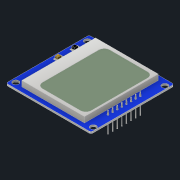
# Autodesk Inventor part: Nokia LCD
Saved by Autodesk Inventor 2022 (Build 260153000, 153)
## iProperties
Created: 2020-05-12
Part Number: Nokia LCD
Material: Generic
Document SubType Name: Modeling
Designer: Arrofiq
Density: 1 g/cm^3
Appearance: Aluminum - Polished
Author: Arrofiq
Autodesk Inventor part; units mm, degrees
ref_plane "YZ Plane" through (0, 0, 0) normal (1, 0, 0) x (0, 1, 0)
ref_plane "XZ Plane" through (0, 0, 0) normal (0, 1, 0) x (-1, 0, 0)
ref_plane "XY Plane" through (0, 0, 0) normal (0, 0, 1) x (1, 0, 0)
sketch "Sketch1" plane through (0, 0, 0) normal (0, 1, 0) x (-1, 0, 0)
  line L0 (23, -22.5) -> (-23, -22.5)
  line L1 (-23, -22.5) -> (-23, 22.5)
  line L2 (-23, 22.5) -> (23, 22.5)
  line L3 (23, 22.5) -> (23, -22.5)
  line L4 (23, -22.5) -> (-23, 22.5) construction
  line L5 (-23, -22.5) -> (23, 22.5) construction
  point P0 (0, 0)
  dimension "d0" = 46
  dimension "d1" = 45
  constraints: 12 end point, 2 midpoint, 2 parallel, 1 horizontal, 1 perpendicular
  measures "d0" distance of L1.end L2.end
  measures "d1" distance of L0.end L1.end
extrude "Extrusion1" add sketch "Sketch1" along normal mid plane 1
sketch "Sketch2" plane through (0, 0.5, 0) normal (0, 1, 0) x (1, 0, 0)
  line L0 (-17, 20) -> (17, 20)
  line L1 (17, 20) -> (17, -20)
  line L2 (17, -20) -> (-17, -20)
  line L3 (-17, -20) -> (-17, 20)
  line L4 (-17, 20) -> (17, -20) construction
  line L5 (17, 20) -> (-17, -20) construction
  line L6 (23, -22.5) -> (23, 22.5) projected
  line L7 (-23, 22.5) -> (-23, -22.5) projected
  point P0 (0, 0)
  point P1 (0, 0)
  point P2 (0, 0)
  dimension "d4" = 34
  dimension "d5" = 40
  dimension "d8" = 6
  dimension "d9" = 6
  constraints: 12 end point, 3 midpoint, 2 parallel, 1 coincident, 1 horizontal, 1 perpendicular
  measures "d4" distance of L1.end L2.end
  measures "d5" distance of L0.end L1.end
  measures "d8" distance between parallel lines of L6 L1
  measures "d9" distance between parallel lines of L7 L3
extrude "Extrusion2" add sketch "Sketch2" along normal blind 3
sketch "Sketch3" plane through (0, 3.5, 0) normal (0, 1, 0) x (1, 0, 0)
  line L0 (-10.5, 18.25) -> (16, 18.25)
  line L1 (16, 18.25) -> (16, -18.25)
  line L2 (16, -18.25) -> (-10.5, -18.25)
  line L3 (-10.5, -18.25) -> (-10.5, 18.25)
  line L4 (-10.5, 18.25) -> (16, -18.25) construction
  line L5 (16, 18.25) -> (-10.5, -18.25) construction
  line L6 (17, -20) -> (17, 20) projected
  point P0 (2.75, 0)
  dimension "d10" = 26.5
  dimension "d11" = 36.5
  dimension "d13" = 1
  constraints: 12 end point, 2 midpoint, 2 parallel, 1 horizontal, 1 perpendicular
  measures "d10" distance of L1.end L2.end
  measures "d11" distance of L0.end L1.end
  measures "d13" distance between parallel lines of L6 L1
extrude "Extrusion3" cut sketch "Sketch3" against normal blind 0.05
sketch "Sketch4" plane through (0, 0.5, 0) normal (0, 1, 0) x (1, 0, 0)
  circle A0 centre (21.3, 19.3) radius 1.6
  line L0 (23, 22.5) -> (-23, 22.5) projected
  line L1 (23, -22.5) -> (23, 22.5) projected
  circle A1 centre (-20.7, 19.3) radius 1.6
  line L2 (-23, 22.5) -> (-23, -22.5) projected
  circle A2 centre (-20.7, -19.5) radius 1.6
  line L3 (-23, -22.5) -> (23, -22.5) projected
  circle A3 centre (21.3, -19.5) radius 1.6
  point P0 (0, 0)
  dimension "d16" = 3.2
  dimension "d19" = 3.2
  dimension "d22" = 3.2
  dimension "d23" = 2.3
  dimension "d24" = 3
  dimension "d25" = 3.2
  dimension "d84" = 38.8
  dimension "d85" = 42
  constraints: 4 centre point, 2 horizontal alignment, 2 vertical alignment
  measures "d16" diameter of A0
  measures "d19" diameter of A1
  measures "d22" diameter of A2
  measures "d23" distance from line of L2 A2.centre
  measures "d24" distance from line of L3 A2.centre
  measures "d25" diameter of A3
  measures "d84" distance of A1.centre A2.centre
  measures "d85" distance of A2.centre A3.centre
extrude "Extrusion4" cut sketch "Sketch4" against normal up to next contours A0 | A1 | A2 | A3
sketch "Sketch5" plane through (0, 0.5, 0) normal (0, 1, 0) x (1, 0, 0)
  circle A0 centre (19.5, -9.75) radius 0.25
  line L0 (-23, 22.5) -> (-23, -22.5) projected
  line L1 (23, -22.5) -> (23, 22.5) projected
  line L2 (-23, -22.5) -> (23, -22.5) projected
  point P0 (0, 0)
  dimension "d32" = 0.5
  dimension "d33" = 3.5
  dimension "d34" = 12.75
  constraints: 1 centre point
  measures "d32" diameter of A0
  measures "d33" distance from line of L1 A0.centre
  measures "d34" distance from line of L2 A0.centre
extrude "Extrusion5" cut sketch "Sketch5" against normal up to next
pattern_linear "Rectangular Pattern1" count 8 spacing 2.5 along (0, 0, -1) of "Extrusion5"
fillet "Fillet1" radius 1 4 edges at (-23, 0, -22.5) (-23, 0, 22.5) (23, 0, 22.5) (23, 0, -22.5)
fillet "Fillet2" radius 3 4 edges at (16, 3.475, 18.25) (16, 3.475, -18.25) (-10.5, 3.475, -18.25) (-10.5, 3.475, 18.25)
sketch "Sketch7" plane through (0, 0.5, 0) normal (0, 1, 0) x (1, 0, 0)
  line L0 (-21.5, 5.5) -> (-20, 5.5)
  line L1 (-20, 5.5) -> (-20, 1.5)
  line L2 (-20, 1.5) -> (-21.5, 1.5)
  line L3 (-21.5, 1.5) -> (-21.5, 5.5)
  line L4 (-21.5, 5.5) -> (-20, 1.5) construction
  line L5 (-20, 5.5) -> (-21.5, 1.5) construction
  line L6 (-23, 21.5) -> (-23, -21.5) projected
  line L7 (22, 22.5) -> (-22, 22.5) projected
  line L8 (-21.5, 14.5) -> (-20, 14.5)
  line L9 (-20, 14.5) -> (-20, 10.5)
  line L10 (-20, 10.5) -> (-21.5, 10.5)
  line L11 (-21.5, 10.5) -> (-21.5, 14.5)
  line L12 (-21.5, 14.5) -> (-20, 10.5) construction
  line L13 (-20, 14.5) -> (-21.5, 10.5) construction
  point P0 (0, 0)
  point P1 (-20.75, 3.5)
  point P2 (-20.75, 12.5)
  dimension "d45" = 1.5
  dimension "d46" = 4
  dimension "d49" = 3
  dimension "d50" = 21
  dimension "d51" = 1.5
  dimension "d52" = 12
  constraints: 24 end point, 4 midpoint, 4 parallel, 2 collinear, 2 horizontal, 2 perpendicular
  measures "d45" distance of L1.end L2.end
  measures "d46" distance of L0.end L1.end
  measures "d49" distance between parallel lines of L6 L1
  measures "d50" distance between parallel lines of L7 L2
  measures "d51" distance of L9.end L10.end
  measures "d52" distance between parallel lines of L7 L10
extrude "Extrusion6" add sketch "Sketch7" along normal blind 0.05
sketch "Sketch8" plane through (0, 0.55, 0) normal (0, 1, 0) x (1, 0, 0)
  line L0 (-21.5, 2.5) -> (-20, 2.5)
  line L1 (-20, 2.5) -> (-20, 4.5)
  line L2 (-20, 4.5) -> (-21.5, 4.5)
  line L3 (-21.5, 4.5) -> (-21.5, 2.5)
  line L4 (-20, 1.5) -> (-20, 5.5) projected
  line L5 (-21.5, 5.5) -> (-21.5, 1.5) projected
  line L6 (-21.5, 1.5) -> (-20, 1.5) projected
  line L7 (-20, 5.5) -> (-21.5, 5.5) projected
  line L8 (-21.5, 11.5) -> (-20, 11.5)
  line L9 (-20, 11.5) -> (-20, 13.5)
  line L10 (-20, 13.5) -> (-21.5, 13.5)
  line L11 (-21.5, 13.5) -> (-21.5, 11.5)
  line L12 (-21.5, 14.5) -> (-21.5, 10.5) projected
  line L13 (-20, 10.5) -> (-20, 14.5) projected
  line L14 (-21.5, 10.5) -> (-20, 10.5) projected
  point P0 (0, 0)
  dimension "d53" = 2
  dimension "d54" = 1
  dimension "d55" = 1
  dimension "d56" = 2
  dimension "d57" = 1
  constraints: 16 end point, 4 collinear, 4 parallel, 2 horizontal, 2 perpendicular
  measures "d53" distance between parallel lines of L2 L0
  measures "d54" distance between parallel lines of L6 L0
  measures "d55" distance between parallel lines of L7 L2
  measures "d56" distance between parallel lines of L8 L10
  measures "d57" distance between parallel lines of L14 L8
extrude "Extrusion7" add sketch "Sketch8" along normal blind 1 contours L3 L2 L1 L0 | L11 L10 L9 L8
fillet "Fillet3" radius 0.25 4 edges at (-20.75, 1.55, -2.5) (-20.75, 1.55, -4.5) (-20.75, 1.55, -11.5) (-20.75, 1.55, -13.5)
sketch "Sketch9" plane through (0, -0.5, 0) normal (0, -1, 0) x (1, 0, 0)
  circle A0 centre (19.5, -7.75) radius 0.25 projected
  circle A1 centre (19.5, -5.25) radius 0.25 projected
  circle A2 centre (19.5, -2.75) radius 0.25 projected
  circle A3 centre (19.5, -0.25) radius 0.25 projected
  circle A4 centre (19.5, 2.25) radius 0.25 projected
  circle A5 centre (19.5, 4.75) radius 0.25 projected
  circle A6 centre (19.5, 7.25) radius 0.25 projected
  circle A7 centre (19.5, 9.75) radius 0.25 projected
  circle A8 centre (-20.7, 19.5) radius 1.6 projected
  circle A9 centre (21.3, -19.3) radius 1.6 projected
  circle A10 centre (-20.7, -19.3) radius 1.6 projected
  circle A11 centre (21.3, 19.5) radius 1.6 projected
  arc A12 (22, -22.5) -> (23, -21.5) centre (22, -21.5) ccw projected
  line L0 (23, -21.5) -> (23, 21.5) projected
  arc A13 (23, 21.5) -> (22, 22.5) centre (22, 21.5) ccw projected
  line L1 (22, 22.5) -> (-22, 22.5) projected
  arc A14 (-22, 22.5) -> (-23, 21.5) centre (-22, 21.5) ccw projected
  line L2 (-23, 21.5) -> (-23, -21.5) projected
  arc A15 (-23, -21.5) -> (-22, -22.5) centre (-22, -21.5) ccw projected
  line L3 (-22, -22.5) -> (22, -22.5) projected
  circle A16 centre (19.5, 9.75) radius 1.25
  circle A17 centre (19.5, 7.25) radius 0.25 projected
  point P0 (0, 0)
  dimension "d61" = 2.5
  constraints: 1 centre point, 1 coincident
  measures "d61" diameter of A16
extrude "Extrusion8" add sketch "Sketch9" along normal blind 2 contours A7 | A16
pattern_linear "Rectangular Pattern2" count 8 spacing 2.5 along (0, 0, -1) of "Extrusion8"
sketch "Sketch10" plane through (19.5, -2.5, 9.75) normal (0, -1, 0) x (1, 0, 0)
  circle A0 centre (0, 0) radius 0.25
  point P0 (-19.5, -9.75)
  dimension "d68" = 0.5
  constraints: 1 centre point
  measures "d68" diameter of A0
extrude "Extrusion9" add sketch "Sketch10" along normal blind 6 and the other way blind 5
pattern_linear "Rectangular Pattern3" count 8 spacing 2.5 along (0, 0, -1) of "Extrusion9"
draft "FaceDraft1" angle 5 pull direction (0, 1, 0) faces at (19.5101, 1.8333, 9.9998) fixed edges at (19.25, 2.5, 9.75)
draft "FaceDraft2" angle 5 pull direction (0, 1, 0) faces at (19.5101, 1.8333, 7.4998) fixed edges at (19.25, 2.5, 7.25)
draft "FaceDraft3" angle 5 pull direction (0, 1, 0) faces at (19.5101, 1.8333, 4.9998) fixed edges at (19.25, 2.5, 4.75)
draft "FaceDraft4" angle 5 pull direction (0, 1, 0) faces at (19.5101, 1.8333, 2.4998) fixed edges at (19.25, 2.5, 2.25)
draft "FaceDraft5" angle 5 pull direction (0, 1, 0) faces at (19.5101, 1.8333, -0.0002) fixed edges at (19.25, 2.5, -0.25)
draft "FaceDraft6" angle 5 pull direction (0, 1, 0) faces at (19.5101, 1.8333, -2.5002) fixed edges at (19.25, 2.5, -2.75)
draft "FaceDraft7" angle 5 pull direction (0, 1, 0) faces at (19.5101, 1.8333, -5.0002) fixed edges at (19.25, 2.5, -5.25)
draft "FaceDraft8" angle 5 pull direction (0, 1, 0) faces at (19.5101, 1.8333, -7.5002) fixed edges at (19.25, 2.5, -7.75)
equation "\"d19\" = d16"
equation "\"d22\" = d19"
equation "\"d25\" = d22"
equation "\"d51\" = d45"
equation "\"d56\" = d53"
body "Solid1"
